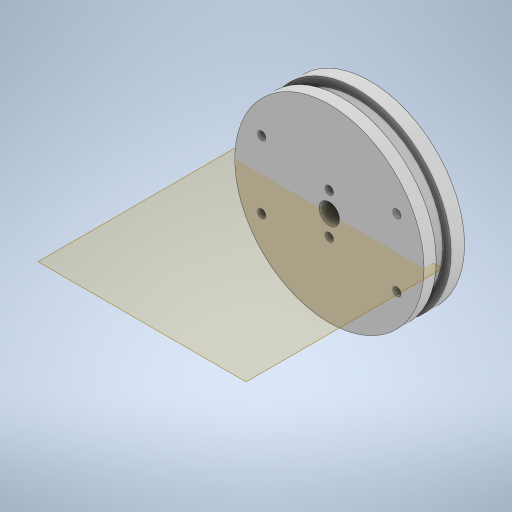
# Autodesk Inventor part: base-top-plate
Saved by Autodesk Inventor 2024 (Build 280153000, 153)
## iProperties
Created: 2024-02-08
Part Number: base-top-plate
Material: Generic
Document SubType Name: Modeling
Designer: MaartenGeorgesBuelen
Density: 1 g/cm^3
Appearance: Default
Sheet Metal Rule: Default
Author: MaartenGeorgesBuelen
## iProperties of the stored document base-top-plate_3DPrint.ipt
Created: 2024-02-09
Part Number: base-top-plate_3DPrint
Material: Generic
Document SubType Name: Modeling
Designer: MaartenGeorgesBuelen
Density: 1 g/cm^3
Appearance: Default
Author: MaartenGeorgesBuelen
Autodesk Inventor part; units mm, degrees
ref_plane "YZ Plane" through (0, 0, 0) normal (1, 0, 0) x (0, 1, 0)
ref_plane "XZ Plane" through (0, 0, 0) normal (0, 1, 0) x (-1, 0, 0)
ref_plane "XY Plane" through (0, 0, 0) normal (0, 0, 1) x (1, 0, 0)
ref_plane "Work Plane1" through (-40, 0, 12) normal (0, 1, 0) x (1, 0, 0)
sketch "Sketch2" plane through (-40, 0, 12) normal (0, 1, 0) x (1, 0, 0)
  line L0 (-30, 12) -> (110, 12) projected
  line L1 (40, 12) -> (40, 42)
  line L2 (40, 42) -> (110, 42)
  line L3 (110, 42) -> (110, 12)
  line L4 (110, 32) -> (104, 32)
  line L5 (104, 32) -> (104, 21)
  line L6 (104, 21) -> (110, 21)
  line L7 (110, 12) -> (40, 12)
  line L8 (40, 12) -> (40, 7)
  line L9 (40, 7) -> (110, 7)
  line L10 (110, 7) -> (110, 12)
  dimension "d3" = 30
  dimension "d4" = 10
  dimension "d5" = 11
  dimension "d6" = 6
  dimension "d17" = 5
  constraints: 20 end point, 3 horizontal, 3 perpendicular, 2 parallel, 2 point on line, 2 vertical
  measures "d3" distance of L1.start L1.end
  measures "d4" distance between parallel lines of L2 L4
  measures "d5" distance of L4.end L5.end
  measures "d6" distance of L5.end L6.end
  measures "d17" distance of L8.end L7.end
revolve "Revolution1" add sketch "Sketch2" angle 360 about axis through (0, 0, 0) along (0, 0, -1) contours L1 L2 L3 L4 L5 L6 L0
sketch "Sketch3" plane through (0, 0, 0) normal (0, 0, 1) x (1, 0, 0)
  circle A0 centre (0, 0) radius 7.5
  dimension "d11" = 15
  constraints: 1 centre point, 1 coincident
  measures "d11" diameter of A0
sketch "Sketch4" plane through (0, 0, 0) normal (0, 0, 1) x (1, 0, 0)
  circle A0 centre (50, 25) radius 2.05 projected
  circle A1 centre (-50, -25) radius 2.05 projected
  circle A2 centre (0, 15) radius 2.05 projected
  circle A3 centre (50, -25) radius 2.05 projected
  circle A4 centre (0, -15) radius 2.05 projected
  circle A5 centre (-50, 25) radius 2.05 projected
  line L0 (-40, 55) -> (40, 55) projected
  line L1 (40, 25) -> (40, 55) projected
  line L2 (40, 25) -> (-40, 25) projected
  line L3 (-40, 55) -> (-40, 25) projected
  line L4 (-40, -31) -> (40, -31) projected
  line L5 (40, -57.4456) -> (40, -31) projected
  arc A6 (40, -57.4456) -> (-40, -57.4456) centre (0, 0) ccw projected
  line L6 (-40, -31) -> (-40, -57.4456) projected
  circle A7 centre (-50, 25) radius 3
  circle A8 centre (-50, -25) radius 3
  circle A9 centre (0, -15) radius 3
  circle A10 centre (0, 15) radius 3
  circle A11 centre (50, 25) radius 3
  circle A12 centre (50, -25) radius 3
  dimension "d8" = 6
  constraints: 6 centre point, 6 coincident, 5 equal radius
  measures "d8" diameter of A7
extrude "Extrusion2" cut sketch "Sketch4" against normal through all contours A0 | A1 | A2 | A3 | A4 | A5 | A7 | A8 | A9 | A10 | A11 | A12
extrude "Extrusion3" cut sketch "Sketch3" against normal blind 11
sketch "Sketch5" plane through (0, 0, -11) normal (0, 0, 1) x (1, 0, 0)
  circle A0 centre (0, 0) radius 2.75
  dimension "d14" = 5.5
  constraints: 1 centre point, 1 coincident
  measures "d14" diameter of A0
extrude "Extrusion4" cut sketch "Sketch5" against normal through all
sketch "Sketch6" plane through (0, 0, 0) normal (0, 0, 1) x (1, 0, 0)
  point P0 (0, 0)
equation "\"BendRadius\" = Thickness"
equation "\"BendReliefWidth\" = Thickness"
equation "\"BendReliefDepth\" = 0.5 * Thickness"
equation "\"CornerReliefSize\" = 4 * Thickness"
equation "\"MinimumRemnant\" = 2 * Thickness"
equation "\"TransitionRadius\" = BendRadius"
equation "\"JacobiRadiusSize\" = BendRadius"
equation "\"GapSize\" = Thickness"
equation "\"Thickness\" = 3.048"
body "Solid2"
